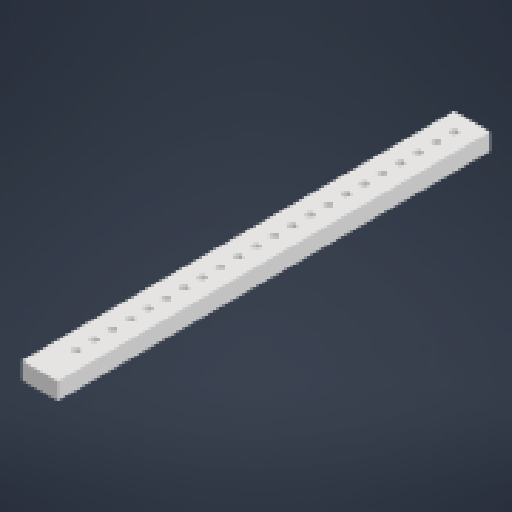
# Autodesk Inventor part: pincer2.0
Saved by Autodesk Inventor 2023 (Build 270158000, 158)
## iProperties
Created: 2023-01-24
Part Number: pincer2.0
Material: Generic
Document SubType Name: Modeling
Designer: Blank Slate
Density: 1 g/cm^3
Appearance: Default
Author: Blank Slate
Autodesk Inventor part; units mm, degrees
ref_plane "YZ Plane" through (0, 0, 0) normal (1, 0, 0) x (0, 1, 0)
ref_plane "XZ Plane" through (0, 0, 0) normal (0, 1, 0) x (-1, 0, 0)
ref_plane "XY Plane" through (0, 0, 0) normal (0, 0, 1) x (1, 0, 0)
sketch "Sketch1" plane through (0, 0, 0) normal (0, 1, 0) x (-1, 0, 0)
  line L0 (0, 0) -> (-25.4, 0)
  line L1 (-25.4, 0) -> (-25.4, -304.8)
  line L2 (-25.4, -304.8) -> (0, -304.8)
  line L3 (0, -304.8) -> (0, 0)
  line L4 (-12.7, 0) -> (-12.7, -304.8) construction
  line L5 (-12.7, 0) -> (-12.7, -25.4)
  line L6 (-12.7, 0) -> (12.7, 0) construction
  circle A0 centre (-12.7, -25.4) radius 2.3813
  circle A1 centre (-12.7, -38.1) radius 2.3813
  circle A2 centre (-12.7, -50.8) radius 2.3813
  circle A3 centre (-12.7, -63.5) radius 2.3813
  circle A4 centre (-12.7, -76.2) radius 2.3813
  circle A5 centre (-12.7, -88.9) radius 2.3813
  circle A6 centre (-12.7, -101.6) radius 2.3813
  circle A7 centre (-12.7, -114.3) radius 2.3813
  circle A8 centre (-12.7, -127) radius 2.3813
  circle A9 centre (-12.7, -139.7) radius 2.3813
  circle A10 centre (-12.7, -152.4) radius 2.3813
  circle A11 centre (-12.7, -165.1) radius 2.3813
  circle A12 centre (-12.7, -177.8) radius 2.3813
  circle A13 centre (-12.7, -190.5) radius 2.3813
  circle A14 centre (-12.7, -203.2) radius 2.3813
  circle A15 centre (-12.7, -215.9) radius 2.3813
  circle A16 centre (-12.7, -228.6) radius 2.3813
  circle A17 centre (-12.7, -241.3) radius 2.3813
  circle A18 centre (-12.7, -254) radius 2.3813
  circle A19 centre (-12.7, -266.7) radius 2.3813
  circle A20 centre (-12.7, -279.4) radius 2.3813
  circle A21 centre (-12.7, -292.1) radius 2.3813
  dimension "d0" = 25.4
  dimension "d1" = 304.8
  dimension "d2" = 25.4
  dimension "d3" = 90
  dimension "d4" = 4.7625
  dimension "d16" = 12.7
  constraints: 22 centre point, 22 coincident, 14 end point, 2 horizontal, 2 midpoint, 2 parallel, 2 perpendicular, 1 collinear, 1 vertical, 63 other
  measures "d0" distance of L2.end L1.end
  measures "d1" distance of L1.end L0.end
  measures "d2" distance of L4.start L5.end
  measures "d3" angle of L5 L6
  measures "d4" diameter of A0
  measures "d16" distance of L5.end point (-12.7, -38.1)
extrude "Extrusion2" add sketch "Sketch1" along normal blind 11.938
body "Solid2"
